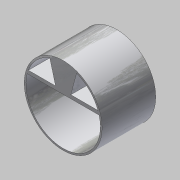
# Autodesk Inventor part: BA001
Saved by Autodesk Inventor 2017 (Build 210142000, 142)
## iProperties
Created: 2017-06-05
Part Number: BA001
Material: ABS Plastic
Document SubType Name: Modeling
Designer: Zach
Density: 1.06 g/cm^3
Appearance: CR White
Mass: 13888.3 g
Surface Area: 14518.4 cm^2
Volume: 13102.2 cm^3
Author: Zach
Autodesk Inventor part; units mm, degrees
ref_plane "YZ Plane" through (0, 0, 0) normal (1, 0, 0) x (0, 1, 0)
ref_plane "XZ Plane" through (0, 0, 0) normal (0, 1, 0) x (-1, 0, 0)
ref_plane "XY Plane" through (0, 0, 0) normal (0, 0, 1) x (1, 0, 0)
sketch "Sketch1" plane through (0, 0, 0) normal (0, 0, 1) x (1, 0, 0)
  circle A0 centre (0, 0) radius 225
  dimension "d0" = 450
  constraints: 1 centre point, 1 coincident
  measures "d0" diameter of A0
extrude "Extrusion1" add sketch "Sketch1" along normal blind 10
sketch "Sketch2" plane through (0, 0, 10) normal (0, 0, 1) x (1, 0, 0)
  circle A0 centre (0, 0) radius 225
  circle A1 centre (0, 0) radius 215
  dimension "d3" = 450
  dimension "d4" = 10
  constraints: 2 centre point, 1 coincident
  measures "d3" diameter of A0
  measures "d4" radial gap between concentric circles of A0 A1
extrude "Extrusion2" add sketch "Sketch2" along normal blind 300
sketch "Sketch5" plane through (0, 0, 10) normal (0, 0, 1) x (1, 0, 0)
  line L0 (-80, 210.2974) -> (80, 210.2974)
  line L1 (80, 210.2974) -> (38.589, 55.7493)
  line L2 (-80, 210.2974) -> (-38.589, 55.7493)
  line L3 (-80, 210.2974) -> (80, 210.2974) construction
  line L4 (-38.589, 55.7493) -> (38.589, 55.7493)
  circle A0 centre (0, 0) radius 225 projected
  dimension "d31" = 160
  dimension "d32" = 160
  dimension "d33" = 75
  dimension "d34" = 160
  dimension "d35" = 75
  constraints: 10 end point, 2 horizontal, 2 point on circle, 1 equal length
  measures "d31" distance of L0.start L0.end
  measures "d32" distance of L0.end L1.end
  measures "d33" angle of L0 L1
  measures "d34" distance of L0.start L2.end
  measures "d35" angle of L2 L3
extrude "Extrusion5" add sketch "Sketch5" along normal blind 300 contours L0 L1 L4 L2
sketch "Sketch6" plane through (0, 0, 10) normal (0, 0, 1) x (1, 0, 0)
  line L0 (-77.3977, 200.5856) -> (-38.589, 55.7493) projected
  line L1 (-38.589, 55.7493) -> (-207.6464, 55.7493)
  arc A0 (-77.3977, 200.5856) -> (77.3977, 200.5856) centre (0, 0) ccw projected
  line L2 (-38.589, 55.7493) -> (38.589, 55.7493) projected
  line L3 (38.589, 55.7493) -> (207.6464, 55.7493)
  line L4 (43.9479, 75.7493) -> (201.2139, 75.7493)
  circle A1 centre (0, 0) radius 225 projected
  line L5 (-43.9479, 75.7493) -> (-211.8656, 75.7493)
  line L6 (-43.9479, 75.7493) -> (-38.589, 55.7493)
  line L7 (43.9479, 75.7493) -> (38.589, 55.7493)
  arc A2 (207.6464, 55.7493) -> (201.2139, 75.7493) centre (0, 0) ccw
  arc A3 (-201.2139, 75.7493) -> (-207.6464, 55.7493) centre (0, 0) ccw
  line L8 (38.589, 55.7493) -> (77.3977, 200.5856) projected
  dimension "d38" = 20
  constraints: 13 end point, 7 point on circle, 6 point on line, 2 centre point, 2 concentric, 2 horizontal, 2 other
  measures "d38" distance between parallel lines of L1 L5
extrude "Extrusion6" add sketch "Sketch6" along normal blind 300 contours L0 L1 A0 L5 | L7 L4 A0 L3
sketch "Sketch7" plane through (0, 0, 10) normal (0, 0, 1) x (1, 0, 0)
  arc A0 (-77.3977, 200.5856) -> (-201.2139, 75.7493) centre (0, 0) ccw projected
  line L0 (-77.3977, 200.5856) -> (-43.9479, 75.7493) projected
  line L1 (-43.9479, 75.7493) -> (-201.2139, 75.7493) projected
  line L2 (-207.6464, 55.7493) -> (207.6464, 55.7493) projected
  arc A1 (-207.6464, 55.7493) -> (207.6464, 55.7493) centre (0, 0) ccw projected
  line L3 (201.2139, 75.7493) -> (43.9479, 75.7493) projected
  line L4 (43.9479, 75.7493) -> (77.3977, 200.5856) projected
  arc A2 (201.2139, 75.7493) -> (77.3977, 200.5856) centre (0, 0) ccw projected
  line L5 (44.7214, 210.2974) -> (-44.7214, 210.2974) projected
  arc A3 (44.7214, 210.2974) -> (-44.7214, 210.2974) centre (0, 0) ccw projected
  circle A4 centre (0, 0) radius 225 projected
extrude "Extrusion7" add sketch "Sketch7" along normal blind 300 contours L5 A3
body "Solid1"
